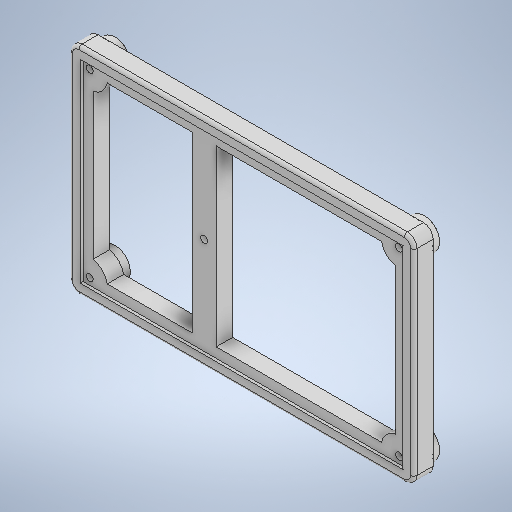
# Autodesk Inventor part: SupportFrame
Saved by Autodesk Inventor 2025 (Build 290162000, 162)
## iProperties
Created: 2026-01-20
Part Number: SupportFrame
Material: Generic
Document SubType Name: Modeling
Designer: tapen
Density: 1 g/cm^3
Appearance: Default
Author: tapen
Autodesk Inventor part; units mm, degrees
ref_plane "YZ Plane" through (0, 0, 0) normal (1, 0, 0) x (0, 1, 0)
ref_plane "XZ Plane" through (0, 0, 0) normal (0, 1, 0) x (-1, 0, 0)
ref_plane "XY Plane" through (0, 0, 0) normal (0, 0, 1) x (1, 0, 0)
sketch "Sketch1" plane through (0, 0, 0) normal (0, 0, 1) x (1, 0, 0)
  line L0 (-103, 63) -> (103, 63)
  line L1 (103, 63) -> (103, -63)
  line L2 (103, -63) -> (-103, -63)
  line L3 (-103, -63) -> (-103, 63)
  line L4 (-103, 63) -> (103, -63) construction
  line L5 (103, 63) -> (-103, -63) construction
  line L6 (-94, 54) -> (94, 54)
  line L7 (94, 54) -> (94, -54)
  line L8 (94, -54) -> (-94, -54)
  line L9 (-94, -54) -> (-94, 54)
  line L10 (-94, 54) -> (94, -54) construction
  line L11 (94, 54) -> (-94, -54) construction
  line L12 (-32.5, 54) -> (-17.5, 54)
  line L13 (-17.5, 54) -> (-17.5, -54)
  line L14 (-17.5, -54) -> (-32.5, -54)
  line L15 (-32.5, -54) -> (-32.5, 54)
  point P0 (0, 0)
  dimension "d0" = 206
  dimension "d1" = 126
  dimension "d2" = 9
  dimension "d3" = 9
  dimension "d4" = 15
  dimension "d5" = 17.5
  constraints: 32 end point, 6 parallel, 4 midpoint, 3 horizontal, 3 perpendicular, 2 point on line
  measures "d0" distance of L1.end L2.end
  measures "d1" distance of L0.end L1.end
  measures "d2" distance between parallel lines of L7 L1
  measures "d3" distance between parallel lines of L2 L8
  measures "d4" distance between parallel lines of L15 L13
  measures "d5" distance from line of L13 point (0, 0)
extrude "Extrusion1" add sketch "Sketch1" along normal blind 12 contours L0 L1 L2 L3 | L6 L13 L8 L15
sketch "Sketch2" plane through (0, 0, 12) normal (0, 0, 1) x (1, 0, 0)
  line L0 (-100.2, 60.2) -> (100.2, 60.2)
  line L1 (100.2, 60.2) -> (100.2, -60.2)
  line L2 (100.2, -60.2) -> (-100.2, -60.2)
  line L3 (-100.2, -60.2) -> (-100.2, 60.2)
  line L4 (-100.2, 60.2) -> (100.2, -60.2) construction
  line L5 (100.2, 60.2) -> (-100.2, -60.2) construction
  point P0 (0, 0)
  dimension "d8" = 200.4
  dimension "d9" = 120.4
  constraints: 12 end point, 2 midpoint, 2 parallel, 1 horizontal, 1 perpendicular
  measures "d8" distance of L1.end L2.end
  measures "d9" distance of L0.end L1.end
extrude "Extrusion2" cut sketch "Sketch2" against normal blind 1.8
sketch "Sketch3" plane through (0, 0, 10.2) normal (0, 0, 1) x (1, 0, 0)
  point P0 (0, 0)
  point P1 (96, 56)
  point P2 (96, -56)
  point P3 (-96, -56)
  point P4 (-96, 56)
  point P5 (-25, 0)
  dimension "d12" = 96
  dimension "d13" = 56
  dimension "d14" = 96
  dimension "d15" = 56
  dimension "d16" = 96
  dimension "d17" = 56
  dimension "d18" = 96
  dimension "d19" = 56
  dimension "d27" = 25
  dimension "d28" = 0
  measures "d12" horizontal distance of point (96, 56) point (0, 0)
  measures "d13" vertical distance of point (0, 0) point (96, 56)
  measures "d14" horizontal distance of point (96, -56) point (0, 0)
  measures "d15" vertical distance of point (0, 0) point (96, -56)
  measures "d16" horizontal distance of point (-96, 56) point (0, 0)
  measures "d17" vertical distance of point (0, 0) point (-96, 56)
  measures "d18" horizontal distance of point (0, 0) point (-96, -56)
  measures "d19" vertical distance of point (0, 0) point (-96, -56)
  measures "d27" distance of point (-25, 0) point (0, 0)
  measures "d28" vertical distance of point (0, 0) point (-25, 0)
hole "Hole1" at (96, 56, 10.2) at (96, -56, 10.2) at (-96, -56, 10.2) at (-96, 56, 10.2) at (-25, 0, 10.2) direction (0, 0, -1) diameter 4.32 end through all
sketch "Sketch4" plane through (0, 0, 0) normal (0, 0, -1) x (-1, 0, 0)
  line L0 (107, -67) -> (-107, -67)
  line L1 (-107, -67) -> (-107, 67)
  line L2 (-107, 67) -> (107, 67)
  line L3 (107, 67) -> (107, -67)
  line L4 (107, -67) -> (-107, 67) construction
  line L5 (-107, -67) -> (107, 67) construction
  line L6 (-103, -63) -> (-103, 63) projected
  line L7 (103, -63) -> (-103, -63)
  line L8 (-103, -63) -> (-103, 63)
  line L9 (-103, 63) -> (103, 63)
  line L10 (103, 63) -> (103, -63)
  line L11 (103, -63) -> (-103, 63) construction
  line L12 (-103, -63) -> (103, 63) construction
  point P0 (0, 0)
  dimension "d29" = 4
  dimension "d30" = 4
  constraints: 24 end point, 4 midpoint, 4 parallel, 2 horizontal, 2 perpendicular
  measures "d29" distance between parallel lines of L9 L2
  measures "d30" distance between parallel lines of L1 L6
extrude "Extrusion3" add sketch "Sketch4" against normal up to surface (12 mm away)
sketch "Sketch5" plane through (0, 0, 10.2) normal (0, 0, 1) x (1, 0, 0)
  circle A0 centre (-96, 56) radius 2.16
  circle A1 centre (-96, 56) radius 11
  line L0 (-107, 67) -> (107, 67)
  line L1 (-32.5, 54) -> (-94, 54)
  line L2 (-94, 54) -> (-94, 45.183346)
  line L3 (-94, -54) -> (-94, 54)
  line L4 (-94, 54) -> (-85.183346, 54)
  circle A2 centre (96, 56) radius 2.16
  circle A3 centre (96, 56) radius 11
  line L5 (94, 54) -> (94, -54)
  line L6 (94, 54) -> (85.183346, 54)
  line L7 (94, 54) -> (-17.5, 54)
  line L8 (94, 54) -> (94, 45.183346)
  circle A4 centre (96, -56) radius 2.16
  circle A5 centre (96, -56) radius 11
  line L9 (107, -67) -> (-107, -67)
  line L10 (94, -54) -> (85.183346, -54)
  line L11 (-17.5, -54) -> (94, -54)
  line L12 (94, -54) -> (94, -45.183346)
  circle A6 centre (-96, -56) radius 2.16
  circle A7 centre (-96, -56) radius 11
  line L13 (-94, -54) -> (-85.183346, -54)
  line L14 (-32.5, -54) -> (-94, -54)
  line L15 (-94, -54) -> (-94, -45.183346)
  point P0 (0, 0)
  constraints: 16 end point, 8 point on circle, 6 point on line, 4 centre point, 4 coincident, 4 tangent, 2 perpendicular
extrude "Extrusion4" add sketch "Sketch5" against normal up to surface (10.2 mm away) contours L2 L1 A1 | A7 L13 L3 | L6 L5 A3 | A5 L5 L10 picked at (-88.385586, 53.158632) picked at (-88.385586, -53.158632) picked at (88.385586, 53.158632) picked at (88.385586, -53.158632)
fillet "Fillet1" radius 6 1 edges at (107, 67, 6)
fillet "Fillet2" radius 6 3 edges at (107, -67, 6) (-107, -67, 6) (-107, 67, 6)
fillet "Fillet3" radius 2 8 edges at (105.2426, 65.2426, 12) (107, 0, 12) (105.2426, -65.2426, 12) (0, -67, 12) (-105.2426, -65.2426, 12) (-107, 0, 12) (-105.2426, 65.2426, 12) (0, 67, 12)
sketch "Sketch9" plane through (0, 0, 0) normal (0, 0, -1) x (-1, 0, 0)
  circle A0 centre (-96, 56) radius 2.16
  arc A1 (-94, 45.183346) -> (-85.183346, 54) centre (-96, 56) ccw
  circle A2 centre (-96, 56) radius 11
  circle A3 centre (96, 56) radius 2.16
  arc A4 (85.183346, 54) -> (94, 45.183346) centre (96, 56) ccw
  circle A5 centre (96, 56) radius 11
  circle A6 centre (96, -56) radius 2.16
  line L0 (85.183346, -54) -> (32.5, -54)
  circle A7 centre (96, -56) radius 11
  circle A8 centre (-96, -56) radius 2.16
  line L1 (-94, -45.183346) -> (-94, 45.183346)
  circle A9 centre (-96, -56) radius 11
  point P0 (0, 0)
  constraints: 4 coincident, 12 other
sketch "Sketch9 outline for Extrusion7" plane through (0, 0, 0) normal (0, 0, -1) x (-1, 0, 0)
  circle A0 centre (-96, -56) radius 11
  circle A1 centre (96, -56) radius 11
  circle A2 centre (96, 56) radius 11
  circle A3 centre (-96, 56) radius 11
extrude "Extrusion7" add sketch "Sketch9 outline for Extrusion7" along normal blind 6 draft -15
sketch "Sketch10" plane through (96, -56, -6) normal (0, 0, -1) x (-1, 0, 0)
  circle A0 centre (0, 0) radius 2.16 projected
  circle A1 centre (0, 0) radius 8.35
  circle A2 centre (0, 112) radius 2.16 projected
  circle A3 centre (0, 112) radius 8.35
  circle A4 centre (192, 112) radius 2.16 projected
  circle A5 centre (192, 112) radius 8.35
  circle A6 centre (192, 0) radius 2.16 projected
  circle A7 centre (192, 0) radius 8.35
  point P0 (96, 56)
  dimension "d53" = 16.7
  dimension "d54" = 16.7
  dimension "d55" = 16.7
  dimension "d56" = 16.7
  constraints: 4 centre point, 4 coincident
  measures "d53" diameter of A1
  measures "d54" diameter of A3
  measures "d55" diameter of A5
  measures "d56" diameter of A7
extrude "Extrusion8" cut sketch "Sketch10" against normal blind 1.5 contours A0 | A1 | A2 | A3 | A4 | A5 | A6 | A7
fillet "Fillet4" radius 0.7 1 edges at (-89.3586, 49.3586, -6)
fillet "Fillet5" radius 0.7 1 edges at (-86.6077, -56, -6)
fillet "Fillet6" radius 0.7 1 edges at (105.3923, -56, -6)
fillet "Fillet7" radius 0.7 1 edges at (97.7077, 65.2358, -6)
equation "\"d3\" = d2"
equation "\"d14\" = d12"
equation "\"d15\" = d13"
equation "\"d16\" = d12"
equation "\"d17\" = d13"
equation "\"d18\" = d12"
equation "\"d19\" = d13"
equation "\"d30\" = d29"
equation "\"d54\" = d53"
equation "\"d55\" = d53"
equation "\"d56\" = d53"
body "Solid1"
